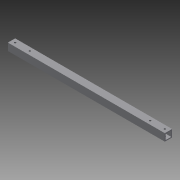
# Autodesk Inventor part: mounting block long
Saved by Autodesk Inventor 2015 SP1 (Build 190203100, 203)
## iProperties
Created: 2015-01-17
Part Number: mounting block long
Material: Generic
Document SubType Name: Modeling
Designer: Jarod
Density: 1 g/cm^3
Appearance: Default
Author: Jarod
Autodesk Inventor part; units mm, degrees
ref_plane "YZ Plane" through (0, 0, 0) normal (1, 0, 0) x (0, 1, 0)
ref_plane "XZ Plane" through (0, 0, 0) normal (0, 1, 0) x (-1, 0, 0)
ref_plane "XY Plane" through (0, 0, 0) normal (0, 0, 1) x (1, 0, 0)
sketch "Sketch1" plane through (0, 0, 0) normal (1, 0, 0) x (0, 1, 0)
  line L0 (0, 0) -> (25.4, 0)
  line L1 (25.4, 0) -> (25.4, -25.4)
  line L2 (25.4, -25.4) -> (0, -25.4)
  line L3 (0, -25.4) -> (0, 0)
  line L4 (3.175, -3.175) -> (22.225, -3.175)
  line L5 (22.225, -3.175) -> (22.225, -22.225)
  line L6 (22.225, -22.225) -> (3.175, -22.225)
  line L7 (3.175, -22.225) -> (3.175, -3.175)
  dimension "d0" = 25.4
  dimension "d1" = 25.4
  dimension "d2" = 19.05
  dimension "d3" = 19.05
  dimension "d4" = 3.175
  dimension "d5" = 3.175
  constraints: 16 end point, 4 parallel, 2 horizontal, 2 perpendicular
  measures "d0" distance of L1.end L2.end
  measures "d1" distance of L0.end L1.end
  measures "d2" distance of L5.end L6.end
  measures "d3" distance of L4.end L5.end
  measures "d4" distance between parallel lines of L0 L4
  measures "d5" distance between parallel lines of L3 L7
extrude "Extrusion1" add sketch "Sketch1" along normal blind 698.5
sketch "Sketch2" plane through (0, 25.4, 0) normal (0, 1, 0) x (1, 0, 0)
  line L0 (0, 0) -> (0, 25.4) projected
  line L1 (0, 0) -> (698.5, 0) projected
  line L2 (698.5, 25.4) -> (698.5, 0) projected
  line L3 (0, 25.4) -> (698.5, 25.4) projected
  point P0 (12.7, 12.7)
  point P1 (88.9, 12.7)
  point P2 (685.8, 12.7)
  point P3 (609.6, 12.7)
  point P4 (139.7, 12.7)
  point P5 (571.5, 12.7)
  point P6 (647.7, 12.7)
  dimension "d8" = 12.7
  dimension "d9" = 88.9
  dimension "d10" = 12.7
  dimension "d11" = 12.7
  dimension "d12" = 12.7
  dimension "d13" = 88.9
  dimension "d14" = 12.7
  dimension "d15" = 12.7
  dimension "d23" = 139.7
  dimension "d24" = 12.7
  dimension "d25" = 127
  dimension "d26" = 12.7
  dimension "d34" = 12.7
  dimension "d35" = 50.8
  measures "d8" distance from line of L0 point (12.7, 12.7)
  measures "d9" distance from line of point (88.9, 12.7) L0
  measures "d10" distance from line of L1 point (12.7, 12.7)
  measures "d11" distance from line of L1 point (88.9, 12.7)
  measures "d12" distance from line of L2 point (685.8, 12.7)
  measures "d13" distance from line of point (609.6, 12.7) L2
  measures "d14" distance from line of L1 point (685.8, 12.7)
  measures "d15" distance from line of L1 point (609.6, 12.7)
  measures "d23" distance from line of L0 point (139.7, 12.7)
  measures "d24" distance from line of L1 point (139.7, 12.7)
  measures "d25" distance from line of point (571.5, 12.7) L2
  measures "d26" distance from line of L1 point (571.5, 12.7)
  measures "d34" distance from line of L1 point (647.7, 12.7)
  measures "d35" distance from line of L2 point (647.7, 12.7)
hole "Hole3" at (12.7, 25.4, -12.7) at (88.9, 25.4, -12.7) at (685.8, 25.4, -12.7) at (609.6, 25.4, -12.7) at (139.7, 25.4, -12.7) at (571.5, 25.4, -12.7) at (647.7, 25.4, -12.7) direction (0, -1, 0) diameter 6.35 end through all
body "Solid1"
